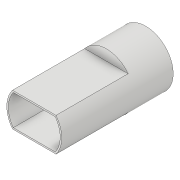
# Autodesk Inventor part: Chassis
Saved by Autodesk Inventor 2017 (Build 210142000, 142)
## iProperties
Created: 2017-03-13
Part Number: Chassis
Material: ABS Plastic
Document SubType Name: Modeling
Designer: zallen
Density: 1.06 g/cm^3
Appearance: Smooth - White
Author: zallen
Autodesk Inventor part; units mm, degrees
ref_plane "YZ Plane" through (0, 0, 0) normal (1, 0, 0) x (0, 1, 0)
ref_plane "XZ Plane" through (0, 0, 0) normal (0, 1, 0) x (-1, 0, 0)
ref_plane "XY Plane" through (0, 0, 0) normal (0, 0, 1) x (1, 0, 0)
sketch "Sketch1" plane through (0, 0, 0) normal (0, 0, 1) x (1, 0, 0)
  circle A0 centre (0, 0) radius 228.6
  dimension "d0" = 457.2
  constraints: 1 centre point, 1 coincident
  measures "d0" diameter of A0
extrude "Extrusion1" add sketch "Sketch1" along normal blind 12.7
sketch "Sketch2" plane through (0, 0, 12.7) normal (0, 0, 1) x (1, 0, 0)
  circle A0 centre (0, 0) radius 228.6
  circle A1 centre (0, 0) radius 215.9
  dimension "d3" = 457.2
  dimension "d4" = 431.8
  constraints: 2 centre point, 2 coincident
  measures "d3" diameter of A0
  measures "d4" diameter of A1
extrude "Extrusion2" add sketch "Sketch2" along normal blind 914.4
sketch "Sketch3" plane through (0, 0, 12.7) normal (0, 0, 1) x (1, 0, 0)
  line L0 (0, -139.7) -> (164.6108, -139.7)
  line L1 (0, -127) -> (174.5961, -127)
  circle A0 centre (0, 0) radius 215.9 projected
  circle A1 centre (0, 0) radius 215.9 projected
  line L2 (0, 127) -> (174.5961, 127)
  line L3 (0, 139.7) -> (164.6108, 139.7)
  line L4 (0, 139.7) -> (-164.6108, 139.7)
  line L5 (0, 127) -> (-174.5961, 127)
  circle A2 centre (0, 0) radius 215.9
  line L6 (0, -127) -> (-174.5961, -127)
  line L7 (0, -139.7) -> (-164.6108, -139.7)
  dimension "d7" = 12.7
  dimension "d8" = 127
  dimension "d9" = 12.7
  dimension "d10" = 127
  constraints: 16 end point, 8 horizontal, 1 centre point, 1 coincident, 9 other
  measures "d7" distance of L1.start L0.start
  measures "d8" distance of point (0, 0) L1.start
  measures "d9" distance of L3.start L2.start
  measures "d10" distance of point (0, 0) L2.start
extrude "Extrusion3" add sketch "Sketch3" along normal blind 914.4 contours L7 A0 L6 L1 L0 | A0 L4 L3 L2 L5
ref_plane "Work Plane3" through (0, 0, 327.1) normal (0, 0, 1) x (1, 0, 0)
sketch "Sketch10" plane through (0, 0, 327.1) normal (0, 0, 1) x (1, 0, 0)
  circle A0 centre (0, 0) radius 228.6 projected
  arc A1 (-164.6108, -139.7) -> (164.6108, -139.7) centre (0, 0) ccw projected
  line L0 (-164.6108, -139.7) -> (-180.9471, -139.7)
  line L1 (164.6108, -139.7) -> (-164.6108, -139.7) projected
  line L2 (164.6108, -139.7) -> (180.9471, -139.7)
  arc A2 (-180.9471, -139.7) -> (180.9471, -139.7) centre (0, 0) ccw
  arc A3 (164.6108, 139.7) -> (-164.6108, 139.7) centre (0, 0) ccw projected
  line L3 (164.6108, 139.7) -> (180.9471, 139.7)
  line L4 (-164.6108, 139.7) -> (164.6108, 139.7) projected
  line L5 (-164.6108, 139.7) -> (-180.9471, 139.7)
  arc A4 (180.9471, 139.7) -> (-180.9471, 139.7) centre (0, 0) ccw
  line L6 (-164.6108, 139.7) -> (164.6108, 139.7)
  line L7 (-164.6108, -139.7) -> (164.6108, -139.7)
  constraints: 12 end point, 9 point on circle, 2 centre point, 2 concentric, 2 horizontal, 1 collinear, 1 parallel, 1 point on line
extrude "Extrusion7" cut sketch "Sketch10" along normal through all contours L3 A3 L5 A0 | A0 L0 A1 L2 | L4 A3 | A1 L1
sketch "Sketch11" plane through (0, 0, 327.1) normal (0, 0, 1) x (1, 0, 0)
  line L0 (-180.9471, -139.7) -> (180.9471, -139.7)
  arc A0 (-180.9471, -139.7) -> (180.9471, -139.7) centre (0, 0) ccw projected
  arc A1 (-180.9471, -139.7) -> (180.9471, -139.7) centre (0, 0) ccw
  line L1 (-180.9471, 139.7) -> (-164.6108, 139.7) projected
  line L2 (-180.9471, 139.7) -> (180.9471, 139.7)
  line L3 (164.6108, 139.7) -> (180.9471, 139.7) projected
  arc A2 (180.9471, 139.7) -> (-180.9471, 139.7) centre (0, 0) ccw
  constraints: 5 point on circle, 4 end point, 2 centre point, 2 point on line, 1 horizontal
extrude "Extrusion8" add sketch "Sketch11" against normal blind 10
body "Solid1"
